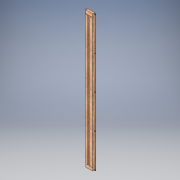
# Autodesk Inventor part: Wiper-Woodconstruction
Saved by Autodesk Inventor 2018.2 (Build 222227000, 227)
## iProperties
Part Number: Wiper-Woodconstruction
Material: Holz (Birke)
Document SubType Name: Modeling
Designer: makerstation
Density: 0.55 g/cm^3
Appearance: Birke - natur - poliert
Author: makerstation
Autodesk Inventor part; units mm, degrees
ref_plane "YZ Plane" through (0, 0, 0) normal (1, 0, 0) x (0, 1, 0)
ref_plane "XZ Plane" through (0, 0, 0) normal (0, 1, 0) x (-1, 0, 0)
ref_plane "XY Plane" through (0, 0, 0) normal (0, 0, 1) x (1, 0, 0)
sketch "Skizze2" plane through (0, 0, 0) normal (0, 1, 0) x (-1, 0, 0)
  line L0 (0, 514) -> (0, -212) construction
  line L1 (-35, 0) -> (35, 0)
  line L2 (35, 0) -> (35, 1020)
  line L3 (35, 1020) -> (-35, 1020)
  line L4 (-35, 1020) -> (-35, 0)
  point P0 (0, 0)
  dimension "breite" = 70
  dimension "laenge" = 1020
  constraints: 10 end point, 2 horizontal, 2 parallel, 2 vertical, 1 perpendicular, 1 other
  measures "breite" distance of L1.start L1.end
  measures "laenge" distance of L3.end L1.start
extrude "Extrusion1" add sketch "Skizze2" along normal blind 4
sketch "Skizze3" plane through (0, 0, 0) normal (0, -1, 0) x (1, 0, 0)
  line L0 (35, 0) -> (-35, 0) projected
  line L1 (35, 1020) -> (35, 0) projected
  line L2 (-35, 1020) -> (35, 1020) projected
  line L3 (-35, 0) -> (-35, 1020) projected
  line L4 (-35, 1020) -> (35, 1020) projected
  line L5 (35, 0) -> (-35, 0) projected
  line L6 (-25, 1020) -> (25, 1020)
  line L7 (25, 1020) -> (25, 0)
  line L8 (25, 0) -> (-25, 0)
  line L9 (-25, 0) -> (-25, 1020)
  line L10 (0, 1159.0325) -> (0, -216) construction
  point P0 (0, 0)
  dimension "d4" = 50
  constraints: 10 end point, 3 parallel, 2 point on line, 1 horizontal, 1 perpendicular, 1 vertical, 1 other
  measures "d4" distance of L8.end L7.end
extrude "Extrusion2" add sketch "Skizze3" along normal blind 14 contours L0 L9 L2 L7
sketch "Skizze4" plane through (0, -14, 0) normal (0, -1, 0) x (1, 0, 0)
  line L0 (-25, 1020) -> (-25, 0) projected
  line L1 (-25, 0) -> (25, 0) projected
  line L2 (25, 0) -> (25, 1020) projected
  line L3 (25, 1020) -> (-25, 1020) projected
  line L4 (-8.5, 995) -> (8.5, 995)
  line L5 (8.5, 995) -> (8.5, 25)
  line L6 (8.5, 25) -> (-8.5, 25)
  line L7 (-8.5, 25) -> (-8.5, 995)
  line L8 (0, -47) -> (0, 1281) construction
  line L9 (-397, 510) -> (541, 510) construction
  line L10 (35, 1020) -> (35, 0) projected
  line L11 (-25, 0) -> (25, 0)
  line L12 (25, 0) -> (25, 25)
  line L13 (25, 25) -> (-25, 25)
  line L14 (-25, 25) -> (-25, 0)
  line L15 (-25, 1020) -> (25, 1020)
  line L16 (25, 1020) -> (25, 995)
  line L17 (25, 995) -> (-25, 995)
  line L18 (-25, 995) -> (-25, 1020)
  line L19 (-24, 1) -> (26, 1)
  line L20 (26, 1021) -> (-24, 1021)
  line L21 (-7.5, 996) -> (9.5, 996)
  line L22 (9.5, 26) -> (-7.5, 26)
  line L23 (-24, 1) -> (26, 1)
  line L24 (26, 1) -> (26, 26)
  line L25 (26, 26) -> (-24, 26)
  line L26 (-24, 26) -> (-24, 1)
  line L27 (-24, 1021) -> (26, 1021)
  line L28 (26, 1021) -> (26, 996)
  line L29 (26, 996) -> (-24, 996)
  line L30 (-24, 996) -> (-24, 1021)
  point P0 (0, 0)
  point P1 (1, 1)
  point P2 (36, 1021)
  point P3 (36, 1)
  dimension "d8" = 25
  dimension "d9" = 510
  dimension "d10" = 35
  dimension "d11" = 17
  dimension "d14" = 25
  dimension "d15" = 17
  constraints: 52 end point, 11 parallel, 7 horizontal, 5 perpendicular, 2 point on line, 2 other
  measures "d8" distance between parallel lines of L6 L1
  measures "d9" distance between parallel lines of L9 L1
  measures "d10" distance between parallel lines of L8 L10
  measures "d11" distance of L5.end L6.end
  measures "d14" distance between parallel lines of L22 L19
  measures "d15" distance of L22.start L22.end
extrude "Extrusion3" cut sketch "Skizze4" against normal blind 10 contours L4 L5 L22 L25 L7 | L25 L22 L5 L6 L7
sketch "Skizze6" plane through (0, -14, 0) normal (0, -1, 0) x (1, 0, 0)
  line L0 (-25, 0) -> (25, 0)
  line L1 (25, 1020) -> (-25, 1020)
  line L2 (-8.5, 995) -> (8.5, 995)
  line L3 (8.5, 25) -> (-8.5, 25)
  line L4 (-25, 0) -> (25, 0)
  line L5 (25, 0) -> (25, 25)
  line L6 (25, 25) -> (-25, 25)
  line L7 (-25, 25) -> (-25, 0)
  line L8 (-25, 1020) -> (25, 1020)
  line L9 (25, 1020) -> (25, 995)
  line L10 (25, 995) -> (-25, 995)
  line L11 (-25, 995) -> (-25, 1020)
  point P0 (0, 0)
  point P1 (0, 0)
  point P2 (35, 1020)
  point P3 (35, 0)
  dimension "d16" = 25
  dimension "d17" = 17
  constraints: 24 end point, 5 parallel, 3 horizontal, 2 perpendicular
  measures "d16" distance between parallel lines of L3 L0
  measures "d17" distance of L3.start L3.end
extrude "Extrusion4" cut sketch "Skizze6" against normal blind 3
sketch "Skizze7" plane through (0, 0, 0) normal (0, -1, 0) x (1, 0, 0)
  line L0 (-25, 0) -> (-25, 1020) projected
  line L1 (-35, 1020) -> (-25, 1020) projected
  line L2 (-35, 0) -> (-35, 1020) projected
  line L3 (-25, 0) -> (-35, 0) projected
  line L4 (25, 1020) -> (25, 0) projected
  line L5 (35, 0) -> (25, 0) projected
  line L6 (35, 1020) -> (35, 0) projected
  line L7 (25, 1020) -> (35, 1020) projected
  line L8 (0, 1058) -> (0, -187) construction
  line L9 (-30, 1012) -> (-30, 5) construction
  point P0 (0, 0)
  point P1 (-30, 760.25)
  point P2 (-30, 508.5)
  point P3 (-30, 256.75)
  point P4 (30, 1012)
  point P5 (30, 5)
  point P6 (30, 760.25)
  point P7 (30, 508.5)
  point P8 (30, 256.75)
  dimension "d20" = 5
  dimension "d21" = 8
  dimension "d22" = 5
  dimension "d23" = 5
  dimension "d26" = 251.75
  dimension "d27" = 503.5
  dimension "d28" = 755.25
  constraints: 5 symmetric about line, 4 end point, 2 point on line, 1 midpoint, 1 vertical
  measures "d20" distance from line of L9.start L2
  measures "d21" distance from line of L9.start L1
  measures "d22" distance from line of L3 L9.end
  measures "d23" distance from line of L2 L9.end
  measures "d26" distance of point (-30, 760.25) L9.start
  measures "d27" distance of point (-30, 508.5) L9.start
  measures "d28" distance of point (-30, 256.75) L9.start
hole "Bohrung1" at (-30, 0, 1012) at (-30, 0, 5) at (-30, 0, 760.25) at (-30, 0, 508.5) at (-30, 0, 256.75) at (30, 0, 1012) at (30, 0, 760.25) at (30, 0, 508.5) at (30, 0, 256.75) at (30, 0, 5) direction (0, 1, 0) diameter 8 depth 1
equation "\"d9\" = 0.5 * laenge"
equation "\"d10\" = 0.5 * breite"
